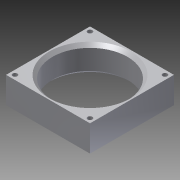
# Autodesk Inventor part: fan
Saved by Autodesk Inventor 2015 (Build 190159000, 159)
## iProperties
Created: 2014-08-15
Part Number: fan
Material: ABS Plastic
Document SubType Name: Modeling
Designer: Christo
Density: 1.06 g/cm^3
Appearance: Smooth - White
Mass: 59.3098 g
Surface Area: 189.057 cm^2
Volume: 55.9526 cm^3
Author: Christo
Autodesk Inventor part; units mm, degrees
ref_plane "YZ Plane" through (0, 0, 0) normal (1, 0, 0) x (0, 1, 0)
ref_plane "XZ Plane" through (0, 0, 0) normal (0, 1, 0) x (-1, 0, 0)
ref_plane "XY Plane" through (0, 0, 0) normal (0, 0, 1) x (1, 0, 0)
sketch "Sketch1" plane through (0, 0, 0) normal (0, 0, 1) x (1, 0, 0)
  line L0 (-40, -40) -> (40, -40)
  line L1 (40, -40) -> (40, 40)
  line L2 (40, 40) -> (-40, 40)
  line L3 (-40, 40) -> (-40, -40)
  point P0 (0, 0)
  point P1 (40, 0)
  point P2 (0, 40)
  dimension "L" = 80
  dimension "d1" = 80
  constraints: 8 end point, 2 midpoint, 2 parallel, 1 horizontal, 1 horizontal alignment, 1 perpendicular, 1 vertical alignment
  measures "L" distance of L1.end L2.end
  measures "d1" distance of L0.end L1.end
extrude "Extrusion1" add sketch "Sketch1" along normal blind 25
sketch "Sketch2" plane through (0, 0, 25) normal (0, 0, 1) x (1, 0, 0)
  line L0 (-35.75, -35.75) -> (35.75, -35.75) construction
  line L1 (35.75, -35.75) -> (35.75, 35.75) construction
  line L2 (35.75, 35.75) -> (-35.75, 35.75) construction
  line L3 (-35.75, 35.75) -> (-35.75, -35.75) construction
  point P0 (0, 0)
  point P1 (-35.75, 0)
  point P2 (0, 35.75)
  dimension "inner" = 71.5
  dimension "d5" = 71.5
  constraints: 8 end point, 4 coincident, 2 midpoint, 2 parallel, 1 horizontal, 1 horizontal alignment, 1 perpendicular, 1 vertical alignment
  measures "inner" distance of L1.end L2.end
  measures "d5" distance of L0.end L1.end
hole "Hole1" at (-35.75, 35.75, 25) at (35.75, 35.75, 25) at (-35.75, -35.75, 25) at (35.75, -35.75, 25) direction (0, 0, -1) diameter 4.5 end through all
sketch "Sketch3" plane through (0, 0, 25) normal (0, 0, 1) x (1, 0, 0)
  point P0 (0, 0)
  point P1 (0, 0)
  constraints: 1 coincident
hole "Hole2" at (0, 0, 25) direction (0, 0, -1) diameter 71.5 end through all
chamfer "Chamfer1" distance 3 angle 45 2 edges at (0, 35.75, 25) (0, 35.75, 0)
equation "\"d1\" = L"
equation "\"d5\" = inner"
body "Solid1"
